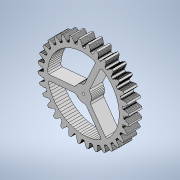
# Autodesk Inventor part: Шестерня 32 зуба
Saved by Autodesk Inventor 2020 (Build 240168000, 168)
## iProperties
Created: 2021-06-13
Part Number: Шестерня 32 зуба
Material: Типовые
Document SubType Name: Modeling
Designer: Антон
Density: 1 g/cm^3
Appearance: По умолчанию
Author: Антон
Autodesk Inventor part; units mm, degrees
(part 1 of 2)
ref_plane "YZ Plane" through (0, 0, 0) normal (1, 0, 0) x (0, 1, 0)
ref_plane "XZ Plane" through (0, 0, 0) normal (0, 1, 0) x (-1, 0, 0)
ref_plane "XY Plane" through (0, 0, 0) normal (0, 0, 1) x (1, 0, 0)
sketch "Эскиз1" plane through (0, 0, 0) normal (0, 0, 1) x (1, 0, 0)
  line L0 (2.3797, 14.7575) -> (2.3075, 14.8611)
  line L1 (2.3075, 14.8611) -> (2.2375, 14.9567)
  line L2 (2.2375, 14.9567) -> (2.1835, 14.9517)
  line L3 (2.1835, 14.9517) -> (2.0746, 14.948)
  line L4 (2.0746, 14.948) -> (1.9648, 14.9497)
  line L5 (1.9648, 14.9497) -> (1.8544, 14.9557)
  line L6 (1.8544, 14.9557) -> (1.6322, 14.9783)
  line L7 (1.6322, 14.9783) -> (1.4083, 15.013)
  line L8 (1.4083, 15.013) -> (1.1833, 15.0583)
  line L9 (1.1833, 15.0583) -> (0.9573, 15.1136)
  line L10 (0.9573, 15.1136) -> (0.7306, 15.178)
  line L11 (0.7306, 15.178) -> (0.5032, 15.2512)
  line L12 (0.5032, 15.2512) -> (0.2756, 15.3329)
  line L13 (0.2756, 15.3329) -> (0.1047, 15.3995)
  line L14 (0.1047, 15.3995) -> (0.0431, 16.0795)
  line L15 (0.0431, 16.0795) -> (0.1992, 16.1757)
  line L16 (0.1992, 16.1757) -> (0.4086, 16.2969)
  line L17 (0.4086, 16.2969) -> (0.619, 16.4098)
  line L18 (0.619, 16.4098) -> (0.8305, 16.5139)
  line L19 (0.8305, 16.5139) -> (1.0429, 16.6088)
  line L20 (1.0429, 16.6088) -> (1.2561, 16.6939)
  line L21 (1.2561, 16.6939) -> (1.4701, 16.7682)
  line L22 (1.4701, 16.7682) -> (1.6846, 16.8303)
  line L23 (1.6846, 16.8303) -> (1.7922, 16.8561)
  line L24 (1.7922, 16.8561) -> (1.8999, 16.8775)
  line L25 (1.8999, 16.8775) -> (2.0077, 16.8934)
  line L26 (2.0077, 16.8934) -> (2.0617, 16.8982)
  line L27 (2.0617, 16.8982) -> (2.1134, 17.0048)
  line L28 (2.1134, 17.0048) -> (2.1657, 17.1197)
  line L29 (2.1657, 17.1197) -> (2.1704, 17.717)
  line L30 (2.1704, 17.717) -> (2.1199, 17.8328)
  line L31 (2.1199, 17.8328) -> (2.0699, 17.9402)
  line L32 (2.0699, 17.9402) -> (2.016, 17.9458)
  line L33 (2.016, 17.9458) -> (1.9084, 17.9634)
  line L34 (1.9084, 17.9634) -> (1.8011, 17.9865)
  line L35 (1.8011, 17.9865) -> (1.694, 18.014)
  line L36 (1.694, 18.014) -> (1.4804, 18.0794)
  line L37 (1.4804, 18.0794) -> (1.2676, 18.1571)
  line L38 (1.2676, 18.1571) -> (1.0557, 18.2455)
  line L39 (1.0557, 18.2455) -> (0.8448, 18.3438)
  line L40 (0.8448, 18.3438) -> (0.635, 18.4512)
  line L41 (0.635, 18.4512) -> (0.4264, 18.5674)
  line L42 (0.4264, 18.5674) -> (0.219, 18.6919)
  line L43 (0.219, 18.6919) -> (0.0644, 18.7905)
  line L44 (0.0644, 18.7905) -> (0.1366, 19.4695)
  line L45 (0.1366, 19.4695) -> (0.3086, 19.5334)
  line L46 (0.3086, 19.5334) -> (0.5375, 19.6114)
  line L47 (0.5375, 19.6114) -> (0.7659, 19.6811)
  line L48 (0.7659, 19.6811) -> (0.9937, 19.7419)
  line L49 (0.9937, 19.7419) -> (1.2205, 19.7936)
  line L50 (1.2205, 19.7936) -> (1.4462, 19.8355)
  line L51 (1.4462, 19.8355) -> (1.6705, 19.8666)
  line L52 (1.6705, 19.8666) -> (1.8932, 19.8857)
  line L53 (1.8932, 19.8857) -> (2.0036, 19.8899)
  line L54 (2.0036, 19.8899) -> (2.1134, 19.8899)
  line L55 (2.1134, 19.8899) -> (2.2223, 19.8845)
  line L56 (2.2223, 19.8845) -> (2.2762, 19.8787)
  line L57 (2.2762, 19.8787) -> (2.3477, 19.9732)
  line L58 (2.3477, 19.9732) -> (2.4214, 20.0756)
  line L59 (2.4214, 20.0756) -> (2.5426, 20.6606)
  line L60 (2.5426, 20.6606) -> (2.5156, 20.7839)
  line L61 (2.5156, 20.7839) -> (2.4875, 20.899)
  line L62 (2.4875, 20.899) -> (2.4357, 20.915)
  line L63 (2.4357, 20.915) -> (2.3336, 20.9533)
  line L64 (2.3336, 20.9533) -> (2.2329, 20.997)
  line L65 (2.2329, 20.997) -> (2.1332, 21.0447)
  line L66 (2.1332, 21.0447) -> (1.9365, 21.1506)
  line L67 (1.9365, 21.1506) -> (1.7429, 21.2683)
  line L68 (1.7429, 21.2683) -> (1.5524, 21.3964)
  line L69 (1.5524, 21.3964) -> (1.3647, 21.5339)
  line L70 (1.3647, 21.5339) -> (1.1799, 21.6802)
  line L71 (1.1799, 21.6802) -> (0.9979, 21.8348)
  line L72 (0.9979, 21.8348) -> (0.8188, 21.9974)
  line L73 (0.8188, 21.9974) -> (0.6864, 22.1243)
  line L74 (0.6864, 22.1243) -> (0.8897, 22.7761)
  line L75 (0.8897, 22.7761) -> (1.0708, 22.8052)
  line L76 (1.0708, 22.8052) -> (1.3106, 22.8371)
  line L77 (1.3106, 22.8371) -> (1.5482, 22.8609)
  line L78 (1.5482, 22.8609) -> (1.7834, 22.8761)
  line L79 (1.7834, 22.8761) -> (2.016, 22.8825)
  line L80 (2.016, 22.8825) -> (2.2456, 22.8795)
  line L81 (2.2456, 22.8795) -> (2.4717, 22.8663)
  line L82 (2.4717, 22.8663) -> (2.6937, 22.8416)
  line L83 (2.6937, 22.8416) -> (2.8029, 22.8242)
  line L84 (2.8029, 22.8242) -> (2.9106, 22.8028)
  line L85 (2.9106, 22.8028) -> (3.0163, 22.7763)
  line L86 (3.0163, 22.7763) -> (3.068, 22.76)
  line L87 (3.068, 22.76) -> (3.1566, 22.8387)
  line L88 (3.1566, 22.8387) -> (3.2489, 22.9249)
  line L89 (3.2489, 22.9249) -> (3.4818, 23.4749)
  line L90 (3.4818, 23.4749) -> (3.4794, 23.6012)
  line L91 (3.4794, 23.6012) -> (3.4743, 23.7196)
  line L92 (3.4743, 23.7196) -> (3.4267, 23.7454)
  line L93 (3.4267, 23.7454) -> (3.334, 23.8028)
  line L94 (3.334, 23.8028) -> (3.2437, 23.8653)
  line L95 (3.2437, 23.8653) -> (3.1553, 23.9316)
  line L96 (3.1553, 23.9316) -> (2.983, 24.0738)
  line L97 (2.983, 24.0738) -> (2.8161, 24.227)
  line L98 (2.8161, 24.227) -> (2.6542, 24.3897)
  line L99 (2.6542, 24.3897) -> (2.497, 24.5612)
  line L100 (2.497, 24.5612) -> (2.3443, 24.7408)
  line L101 (2.3443, 24.7408) -> (2.1959, 24.9279)
  line L102 (2.1959, 24.9279) -> (2.052, 25.1223)
  line L103 (2.052, 25.1223) -> (1.9469, 25.2726)
  line L104 (1.9469, 25.2726) -> (2.2735, 25.8722)
  line L105 (2.2735, 25.8722) -> (2.4568, 25.8655)
  line L106 (2.4568, 25.8655) -> (2.6982, 25.85)
  line L107 (2.6982, 25.85) -> (2.9358, 25.8269)
  line L108 (2.9358, 25.8269) -> (3.1695, 25.796)
  line L109 (3.1695, 25.796) -> (3.3989, 25.7569)
  line L110 (3.3989, 25.7569) -> (3.6234, 25.7092)
  line L111 (3.6234, 25.7092) -> (3.8426, 25.6522)
  line L112 (3.8426, 25.6522) -> (4.0556, 25.5846)
  line L113 (4.0556, 25.5846) -> (4.1593, 25.5462)
  line L114 (4.1593, 25.5462) -> (4.2607, 25.5042)
  line L115 (4.2607, 25.5042) -> (4.3592, 25.4576)
  line L116 (4.3592, 25.4576) -> (4.4068, 25.4315)
  line L117 (4.4068, 25.4315) -> (4.509, 25.4915)
  line L118 (4.509, 25.4915) -> (4.6163, 25.5579)
  line L119 (4.6163, 25.5579) -> (4.9521, 26.052)
  line L120 (4.9521, 26.052) -> (4.9744, 26.1763)
  line L121 (4.9744, 26.1763) -> (4.9925, 26.2934)
  line L122 (4.9925, 26.2934) -> (4.9507, 26.328)
  line L123 (4.9507, 26.328) -> (4.8711, 26.4024)
  line L124 (4.8711, 26.4024) -> (4.7947, 26.4813)
  line L125 (4.7947, 26.4813) -> (4.7209, 26.5636)
  line L126 (4.7209, 26.5636) -> (4.5797, 26.7367)
  line L127 (4.5797, 26.7367) -> (4.4459, 26.9195)
  line L128 (4.4459, 26.9195) -> (4.3189, 27.1107)
  line L129 (4.3189, 27.1107) -> (4.1981, 27.3095)
  line L130 (4.1981, 27.3095) -> (4.0833, 27.5154)
  line L131 (4.0833, 27.5154) -> (3.9744, 27.7279)
  line L132 (3.9744, 27.7279) -> (3.8711, 27.9467)
  line L133 (3.8711, 27.9467) -> (3.7974, 28.1146)
  line L134 (3.7974, 28.1146) -> (4.2346, 28.639)
  line L135 (4.2346, 28.639) -> (4.4131, 28.5966)
  line L136 (4.4131, 28.5966) -> (4.6468, 28.5343)
  line L137 (4.6468, 28.5343) -> (4.8754, 28.4653)
  line L138 (4.8754, 28.4653) -> (5.0986, 28.3894)
  line L139 (5.0986, 28.3894) -> (5.3159, 28.3063)
  line L140 (5.3159, 28.3063) -> (5.5269, 28.2157)
  line L141 (5.5269, 28.2157) -> (5.7307, 28.117)
  line L142 (5.7307, 28.117) -> (5.9264, 28.0092)
  line L143 (5.9264, 28.0092) -> (6.0206, 27.9513)
  line L144 (6.0206, 27.9513) -> (6.1119, 27.8903)
  line L145 (6.1119, 27.8903) -> (6.1994, 27.8254)
  line L146 (6.1994, 27.8254) -> (6.241, 27.7905)
  line L147 (6.241, 27.7905) -> (6.3529, 27.8294)
  line L148 (6.3529, 27.8294) -> (6.4712, 27.8736)
  line L149 (6.4712, 27.8736) -> (6.8968, 28.2927)
  line L150 (6.8968, 28.2927) -> (6.9429, 28.4102)
  line L151 (6.9429, 28.4102) -> (6.9836, 28.5215)
  line L152 (6.9836, 28.5215) -> (6.9494, 28.5636)
  line L153 (6.9494, 28.5636) -> (6.8858, 28.6522)
  line L154 (6.8858, 28.6522) -> (6.8262, 28.7444)
  line L155 (6.8262, 28.7444) -> (6.7699, 28.8395)
  line L156 (6.7699, 28.8395) -> (6.6652, 29.0369)
  line L157 (6.6652, 29.0369) -> (6.5696, 29.2422)
  line L158 (6.5696, 29.2422) -> (6.4824, 29.4546)
  line L159 (6.4824, 29.4546) -> (6.4027, 29.6731)
  line L160 (6.4027, 29.6731) -> (6.3303, 29.8975)
  line L161 (6.3303, 29.8975) -> (6.2649, 30.1272)
  line L162 (6.2649, 30.1272) -> (6.2063, 30.3618)
  line L163 (6.2063, 30.3618) -> (6.1667, 30.5409)
  line L164 (6.1667, 30.5409) -> (6.6979, 30.9699)
  line L165 (6.6979, 30.9699) -> (6.8647, 30.8935)
  line L166 (6.8647, 30.8935) -> (7.0817, 30.7869)
  line L167 (7.0817, 30.7869) -> (7.2925, 30.6746)
  line L168 (7.2925, 30.6746) -> (7.4966, 30.5566)
  line L169 (7.4966, 30.5566) -> (7.6935, 30.4327)
  line L170 (7.6935, 30.4327) -> (7.8827, 30.3027)
  line L171 (7.8827, 30.3027) -> (8.0634, 30.1661)
  line L172 (8.0634, 30.1661) -> (8.2342, 30.0222)
  line L173 (8.2342, 30.0222) -> (8.3154, 29.9471)
  line L174 (8.3154, 29.9471) -> (8.393, 29.8695)
  line L175 (8.393, 29.8695) -> (8.4662, 29.7886)
  line L176 (8.4662, 29.7886) -> (8.5001, 29.7464)
  line L177 (8.5001, 29.7464) -> (8.6175, 29.7626)
  line L178 (8.6175, 29.7626) -> (8.7421, 29.783)
  line L179 (8.7421, 29.783) -> (9.2414, 30.1109)
  line L180 (9.2414, 30.1109) -> (9.3095, 30.2172)
  line L181 (9.3095, 30.2172) -> (9.3711, 30.3185)
  line L182 (9.3711, 30.3185) -> (9.3458, 30.3664)
  line L183 (9.3458, 30.3664) -> (9.3006, 30.4657)
  line L184 (9.3006, 30.4657) -> (9.2603, 30.5677)
  line L185 (9.2603, 30.5677) -> (9.2236, 30.672)
  line L186 (9.2236, 30.672) -> (9.1593, 30.886)
  line L187 (9.1593, 30.886) -> (9.1057, 31.1061)
  line L188 (9.1057, 31.1061) -> (9.0615, 31.3313)
  line L189 (9.0615, 31.3313) -> (9.026, 31.5613)
  line L190 (9.026, 31.5613) -> (8.9988, 31.7954)
  line L191 (8.9988, 31.7954) -> (8.9795, 32.0334)
  line L192 (8.9795, 32.0334) -> (8.9678, 32.275)
  line L193 (8.9678, 32.275) -> (8.9639, 32.4584)
  line L194 (8.9639, 32.4584) -> (9.5686, 32.7755)
  line L195 (9.5686, 32.7755) -> (9.7172, 32.6681)
  line L196 (9.7172, 32.6681) -> (9.9093, 32.5211)
  line L197 (9.9093, 32.5211) -> (10.0941, 32.3698)
  line L198 (10.0941, 32.3698) -> (10.2713, 32.2143)
  line L199 (10.2713, 32.2143) -> (10.4402, 32.0544)
  line L200 (10.4402, 32.0544) -> (10.6004, 31.89)
  line L201 (10.6004, 31.89) -> (10.751, 31.7207)
  line L202 (10.751, 31.7207) -> (10.8905, 31.5463)
  line L203 (10.8905, 31.5463) -> (10.9554, 31.4568)
  line L204 (10.9554, 31.4568) -> (11.0164, 31.3655)
  line L205 (11.0164, 31.3655) -> (11.0724, 31.272)
  line L206 (11.0724, 31.272) -> (11.0975, 31.2239)
  line L207 (11.0975, 31.2239) -> (11.2158, 31.2169)
  line L208 (11.2158, 31.2169) -> (11.342, 31.2126)
  line L209 (11.342, 31.2126) -> (11.8956, 31.4368)
  line L210 (11.8956, 31.4368) -> (11.9832, 31.5278)
  line L211 (11.9832, 31.5278) -> (12.0633, 31.6151)
  line L212 (12.0633, 31.6151) -> (12.0478, 31.667)
  line L213 (12.0478, 31.667) -> (12.0229, 31.7732)
  line L214 (12.0229, 31.7732) -> (12.0032, 31.8812)
  line L215 (12.0032, 31.8812) -> (11.9876, 31.9906)
  line L216 (11.9876, 31.9906) -> (11.9663, 32.213)
  line L217 (11.9663, 32.213) -> (11.9567, 32.4393)
  line L218 (11.9567, 32.4393) -> (11.9573, 32.6689)
  line L219 (11.9573, 32.6689) -> (11.9674, 32.9013)
  line L220 (11.9674, 32.9013) -> (11.9863, 33.1363)
  line L221 (11.9863, 33.1363) -> (12.0138, 33.3735)
  line L222 (12.0138, 33.3735) -> (12.0494, 33.6127)
  line L223 (12.0494, 33.6127) -> (12.0814, 33.7933)
  line L224 (12.0814, 33.7933) -> (12.7363, 33.9864)
  line L225 (12.7363, 33.9864) -> (12.8612, 33.852)
  line L226 (12.8612, 33.852) -> (13.0209, 33.6704)
  line L227 (13.0209, 33.6704) -> (13.1727, 33.486)
  line L228 (13.1727, 33.486) -> (13.316, 33.2989)
  line L229 (13.316, 33.2989) -> (13.4506, 33.1091)
  line L230 (13.4506, 33.1091) -> (13.5756, 32.9166)
  line L231 (13.5756, 32.9166) -> (13.6902, 32.7212)
  line L232 (13.6902, 32.7212) -> (13.793, 32.5228)
  line L233 (13.793, 32.5228) -> (13.8392, 32.4224)
  line L234 (13.8392, 32.4224) -> (13.8813, 32.321)
  line L235 (13.8813, 32.321) -> (13.918, 32.2183)
  line L236 (13.918, 32.2183) -> (13.9332, 32.1663)
  line L237 (13.9332, 32.1663) -> (14.0478, 32.1364)
  line L238 (14.0478, 32.1364) -> (14.1707, 32.1075)
  line L239 (14.1707, 32.1075) -> (14.7575, 32.2194)
  line L240 (14.7575, 32.2194) -> (14.8611, 32.2915)
  line L241 (14.8611, 32.2915) -> (14.9567, 32.3615)
  line L242 (14.9567, 32.3615) -> (14.9517, 32.4155)
  line L243 (14.9517, 32.4155) -> (14.948, 32.5245)
  line L244 (14.948, 32.5245) -> (14.9497, 32.6343)
  line L245 (14.9497, 32.6343) -> (14.9557, 32.7447)
  line L246 (14.9557, 32.7447) -> (14.9783, 32.9669)
  line L247 (14.9783, 32.9669) -> (15.013, 33.1907)
  line L248 (15.013, 33.1907) -> (15.0583, 33.4158)
  line L249 (15.0583, 33.4158) -> (15.1136, 33.6418)
  line L250 (15.1136, 33.6418) -> (15.178, 33.8685)
  line L251 (15.178, 33.8685) -> (15.2512, 34.0958)
  line L252 (15.2512, 34.0958) -> (15.3329, 34.3235)
  line L253 (15.3329, 34.3235) -> (15.3995, 34.4944)
  line L254 (15.3995, 34.4944) -> (16.0795, 34.556)
  line L255 (16.0795, 34.556) -> (16.1757, 34.3998)
  line L256 (16.1757, 34.3998) -> (16.2969, 34.1905)
  line L257 (16.2969, 34.1905) -> (16.4098, 33.9801)
  line L258 (16.4098, 33.9801) -> (16.5139, 33.7686)
  line L259 (16.5139, 33.7686) -> (16.6088, 33.5562)
  line L260 (16.6088, 33.5562) -> (16.6939, 33.343)
  line L261 (16.6939, 33.343) -> (16.7682, 33.129)
  line L262 (16.7682, 33.129) -> (16.8303, 32.9144)
  line L263 (16.8303, 32.9144) -> (16.8561, 32.8069)
  line L264 (16.8561, 32.8069) -> (16.8775, 32.6992)
  line L265 (16.8775, 32.6992) -> (16.8934, 32.5914)
  line L266 (16.8934, 32.5914) -> (16.8982, 32.5374)
  line L267 (16.8982, 32.5374) -> (17.0048, 32.4857)
  line L268 (17.0048, 32.4857) -> (17.1197, 32.4334)
  line L269 (17.1197, 32.4334) -> (17.717, 32.4287)
  line L270 (17.717, 32.4287) -> (17.8328, 32.4792)
  line L271 (17.8328, 32.4792) -> (17.9402, 32.5292)
  line L272 (17.9402, 32.5292) -> (17.9458, 32.5831)
  line L273 (17.9458, 32.5831) -> (17.9634, 32.6907)
  line L274 (17.9634, 32.6907) -> (17.9865, 32.798)
  line L275 (17.9865, 32.798) -> (18.014, 32.9051)
  line L276 (18.014, 32.9051) -> (18.0794, 33.1187)
  line L277 (18.0794, 33.1187) -> (18.1571, 33.3315)
  line L278 (18.1571, 33.3315) -> (18.2455, 33.5433)
  line L279 (18.2455, 33.5433) -> (18.3438, 33.7542)
  line L280 (18.3438, 33.7542) -> (18.4512, 33.9641)
  line L281 (18.4512, 33.9641) -> (18.5674, 34.1727)
  line L282 (18.5674, 34.1727) -> (18.6919, 34.3801)
  line L283 (18.6919, 34.3801) -> (18.7905, 34.5347)
  line L284 (18.7905, 34.5347) -> (19.4695, 34.4624)
  line L285 (19.4695, 34.4624) -> (19.5334, 34.2905)
  line L286 (19.5334, 34.2905) -> (19.6114, 34.0616)
  line L287 (19.6114, 34.0616) -> (19.6811, 33.8332)
  line L288 (19.6811, 33.8332) -> (19.7419, 33.6054)
  line L289 (19.7419, 33.6054) -> (19.7936, 33.3786)
  line L290 (19.7936, 33.3786) -> (19.8355, 33.1529)
  line L291 (19.8355, 33.1529) -> (19.8666, 32.9285)
  line L292 (19.8666, 32.9285) -> (19.8857, 32.7059)
  line L293 (19.8857, 32.7059) -> (19.8899, 32.5954)
  line L294 (19.8899, 32.5954) -> (19.8899, 32.4857)
  line L295 (19.8899, 32.4857) -> (19.8845, 32.3768)
  line L296 (19.8845, 32.3768) -> (19.8787, 32.3229)
  line L297 (19.8787, 32.3229) -> (19.9732, 32.2514)
  line L298 (19.9732, 32.2514) -> (20.0756, 32.1776)
  line L299 (20.0756, 32.1776) -> (20.6606, 32.0565)
  line L300 (20.6606, 32.0565) -> (20.7839, 32.0835)
  line L301 (20.7839, 32.0835) -> (20.899, 32.1116)
  line L302 (20.899, 32.1116) -> (20.915, 32.1634)
  line L303 (20.915, 32.1634) -> (20.9533, 32.2655)
  line L304 (20.9533, 32.2655) -> (20.997, 32.3662)
  line L305 (20.997, 32.3662) -> (21.0447, 32.4659)
  line L306 (21.0447, 32.4659) -> (21.1506, 32.6626)
  line L307 (21.1506, 32.6626) -> (21.2683, 32.8561)
  line L308 (21.2683, 32.8561) -> (21.3964, 33.0467)
  line L309 (21.3964, 33.0467) -> (21.5339, 33.2343)
  line L310 (21.5339, 33.2343) -> (21.6802, 33.4192)
  line L311 (21.6802, 33.4192) -> (21.8348, 33.6011)
  line L312 (21.8348, 33.6011) -> (21.9974, 33.7803)
  line L313 (21.9974, 33.7803) -> (22.1243, 33.9127)
  line L314 (22.1243, 33.9127) -> (22.7761, 33.7093)
  line L315 (22.7761, 33.7093) -> (22.8052, 33.5282)
  line L316 (22.8052, 33.5282) -> (22.8371, 33.2885)
  line L317 (22.8371, 33.2885) -> (22.8609, 33.0509)
  line L318 (22.8609, 33.0509) -> (22.8761, 32.8156)
  line L319 (22.8761, 32.8156) -> (22.8825, 32.5831)
  line L320 (22.8825, 32.5831) -> (22.8795, 32.3535)
  line L321 (22.8795, 32.3535) -> (22.8663, 32.1274)
  line L322 (22.8663, 32.1274) -> (22.8416, 31.9054)
  line L323 (22.8416, 31.9054) -> (22.8242, 31.7962)
  line L324 (22.8242, 31.7962) -> (22.8028, 31.6885)
  line L325 (22.8028, 31.6885) -> (22.7763, 31.5828)
  line L326 (22.7763, 31.5828) -> (22.76, 31.5311)
  line L327 (22.76, 31.5311) -> (22.8387, 31.4425)
  line L328 (22.8387, 31.4425) -> (22.9249, 31.3502)
  line L329 (22.9249, 31.3502) -> (23.4749, 31.1173)
  line L330 (23.4749, 31.1173) -> (23.6012, 31.1197)
  line L331 (23.6012, 31.1197) -> (23.7196, 31.1247)
  line L332 (23.7196, 31.1247) -> (23.7454, 31.1724)
  line L333 (23.7454, 31.1724) -> (23.8028, 31.2651)
  line L334 (23.8028, 31.2651) -> (23.8653, 31.3554)
  line L335 (23.8653, 31.3554) -> (23.9316, 31.4438)
  line L336 (23.9316, 31.4438) -> (24.0738, 31.6161)
  line L337 (24.0738, 31.6161) -> (24.227, 31.783)
  line L338 (24.227, 31.783) -> (24.3897, 31.9449)
  line L339 (24.3897, 31.9449) -> (24.5612, 32.1021)
  line L340 (24.5612, 32.1021) -> (24.7408, 32.2548)
  line L341 (24.7408, 32.2548) -> (24.9279, 32.4031)
  line L342 (24.9279, 32.4031) -> (25.1223, 32.5471)
  line L343 (25.1223, 32.5471) -> (25.2726, 32.6522)
  line L344 (25.2726, 32.6522) -> (25.8722, 32.3256)
  line L345 (25.8722, 32.3256) -> (25.8655, 32.1423)
  line L346 (25.8655, 32.1423) -> (25.85, 31.9009)
  line L347 (25.85, 31.9009) -> (25.8269, 31.6632)
  line L348 (25.8269, 31.6632) -> (25.796, 31.4295)
  line L349 (25.796, 31.4295) -> (25.7569, 31.2002)
  line L350 (25.7569, 31.2002) -> (25.7092, 30.9757)
  line L351 (25.7092, 30.9757) -> (25.6522, 30.7565)
  line L352 (25.6522, 30.7565) -> (25.5846, 30.5435)
  line L353 (25.5846, 30.5435) -> (25.5462, 30.4398)
  line L354 (25.5462, 30.4398) -> (25.5042, 30.3384)
  line L355 (25.5042, 30.3384) -> (25.4576, 30.2399)
  line L356 (25.4576, 30.2399) -> (25.4315, 30.1923)
  line L357 (25.4315, 30.1923) -> (25.4915, 30.0901)
  line L358 (25.4915, 30.0901) -> (25.5579, 29.9827)
  line L359 (25.5579, 29.9827) -> (26.052, 29.647)
  line L360 (26.052, 29.647) -> (26.1763, 29.6247)
  line L361 (26.1763, 29.6247) -> (26.2934, 29.6066)
  line L362 (26.2934, 29.6066) -> (26.328, 29.6483)
  line L363 (26.328, 29.6483) -> (26.4024, 29.728)
  line L364 (26.4024, 29.728) -> (26.4813, 29.8044)
  line L365 (26.4813, 29.8044) -> (26.5636, 29.8782)
  line L366 (26.5636, 29.8782) -> (26.7367, 30.0194)
  line L367 (26.7367, 30.0194) -> (26.9195, 30.1532)
  line L368 (26.9195, 30.1532) -> (27.1107, 30.2802)
  line L369 (27.1107, 30.2802) -> (27.3095, 30.401)
  line L370 (27.3095, 30.401) -> (27.5154, 30.5157)
  line L371 (27.5154, 30.5157) -> (27.7279, 30.6247)
  line L372 (27.7279, 30.6247) -> (27.9467, 30.7279)
  line L373 (27.9467, 30.7279) -> (28.1146, 30.8017)
  line L374 (28.1146, 30.8017) -> (28.639, 30.3644)
  line L375 (28.639, 30.3644) -> (28.5966, 30.186)
  line L376 (28.5966, 30.186) -> (28.5343, 29.9522)
  line L377 (28.5343, 29.9522) -> (28.4653, 29.7236)
  line L378 (28.4653, 29.7236) -> (28.3894, 29.5005)
  line L379 (28.3894, 29.5005) -> (28.3063, 29.2831)
  line L380 (28.3063, 29.2831) -> (28.2157, 29.0722)
  line L381 (28.2157, 29.0722) -> (28.117, 28.8684)
  line L382 (28.117, 28.8684) -> (28.0092, 28.6727)
  line L383 (28.0092, 28.6727) -> (27.9513, 28.5785)
  line L384 (27.9513, 28.5785) -> (27.8903, 28.4872)
  line L385 (27.8903, 28.4872) -> (27.8254, 28.3997)
  line L386 (27.8254, 28.3997) -> (27.7905, 28.3581)
  line L387 (27.7905, 28.3581) -> (27.8294, 28.2462)
  line L388 (27.8294, 28.2462) -> (27.8736, 28.1279)
  line L389 (27.8736, 28.1279) -> (28.2927, 27.7022)
  line L390 (28.2927, 27.7022) -> (28.4102, 27.6561)
  line L391 (28.4102, 27.6561) -> (28.5215, 27.6155)
  line L392 (28.5215, 27.6155) -> (28.5636, 27.6497)
  line L393 (28.5636, 27.6497) -> (28.6522, 27.7133)
  line L394 (28.6522, 27.7133) -> (28.7444, 27.7728)
  line L395 (28.7444, 27.7728) -> (28.8395, 27.8292)
  line L396 (28.8395, 27.8292) -> (29.0369, 27.9339)
  line L397 (29.0369, 27.9339) -> (29.2422, 28.0294)
  line L398 (29.2422, 28.0294) -> (29.4546, 28.1167)
  line L399 (29.4546, 28.1167) -> (29.6731, 28.1964)
  line L400 (29.6731, 28.1964) -> (29.8975, 28.2688)
  line L401 (29.8975, 28.2688) -> (30.1272, 28.3342)
  line L402 (30.1272, 28.3342) -> (30.3618, 28.3928)
  line L403 (30.3618, 28.3928) -> (30.5409, 28.4323)
  line L404 (30.5409, 28.4323) -> (30.9699, 27.9012)
  line L405 (30.9699, 27.9012) -> (30.8935, 27.7344)
  line L406 (30.8935, 27.7344) -> (30.7869, 27.5173)
  line L407 (30.7869, 27.5173) -> (30.6746, 27.3066)
  line L408 (30.6746, 27.3066) -> (30.5566, 27.1025)
  line L409 (30.5566, 27.1025) -> (30.4327, 26.9056)
  line L410 (30.4327, 26.9056) -> (30.3027, 26.7164)
  line L411 (30.3027, 26.7164) -> (30.1661, 26.5357)
  line L412 (30.1661, 26.5357) -> (30.0222, 26.3648)
  line L413 (30.0222, 26.3648) -> (29.9471, 26.2837)
  line L414 (29.9471, 26.2837) -> (29.8695, 26.2061)
  line L415 (29.8695, 26.2061) -> (29.7886, 26.1329)
  line L416 (29.7886, 26.1329) -> (29.7464, 26.0989)
  line L417 (29.7464, 26.0989) -> (29.7626, 25.9816)
  line L418 (29.7626, 25.9816) -> (29.783, 25.857)
  line L419 (29.783, 25.857) -> (30.1109, 25.3577)
  line L420 (30.1109, 25.3577) -> (30.2172, 25.2895)
  line L421 (30.2172, 25.2895) -> (30.3185, 25.228)
  line L422 (30.3185, 25.228) -> (30.3664, 25.2533)
  line L423 (30.3664, 25.2533) -> (30.4657, 25.2984)
  line L424 (30.4657, 25.2984) -> (30.5677, 25.3388)
  line L425 (30.5677, 25.3388) -> (30.672, 25.3755)
  line L426 (30.672, 25.3755) -> (30.886, 25.4397)
  line L427 (30.886, 25.4397) -> (31.1061, 25.4934)
  line L428 (31.1061, 25.4934) -> (31.3313, 25.5376)
  line L429 (31.3313, 25.5376) -> (31.5613, 25.573)
  line L430 (31.5613, 25.573) -> (31.7954, 25.6003)
  line L431 (31.7954, 25.6003) -> (32.0334, 25.6196)
  line L432 (32.0334, 25.6196) -> (32.275, 25.6313)
  line L433 (32.275, 25.6313) -> (32.4584, 25.6352)
  line L434 (32.4584, 25.6352) -> (32.7755, 25.0305)
  line L435 (32.7755, 25.0305) -> (32.6681, 24.8819)
  line L436 (32.6681, 24.8819) -> (32.5211, 24.6898)
  line L437 (32.5211, 24.6898) -> (32.3698, 24.505)
  line L438 (32.3698, 24.505) -> (32.2143, 24.3278)
  line L439 (32.2143, 24.3278) -> (32.0544, 24.1588)
  line L440 (32.0544, 24.1588) -> (31.89, 23.9986)
  line L441 (31.89, 23.9986) -> (31.7207, 23.8481)
  line L442 (31.7207, 23.8481) -> (31.5463, 23.7086)
  line L443 (31.5463, 23.7086) -> (31.4568, 23.6437)
  line L444 (31.4568, 23.6437) -> (31.3655, 23.5827)
  line L445 (31.3655, 23.5827) -> (31.272, 23.5267)
  line L446 (31.272, 23.5267) -> (31.2239, 23.5016)
  line L447 (31.2239, 23.5016) -> (31.2169, 23.3833)
  line L448 (31.2169, 23.3833) -> (31.2126, 23.2571)
  line L449 (31.2126, 23.2571) -> (31.4368, 22.7035)
  line L450 (31.4368, 22.7035) -> (31.5278, 22.6159)
  line L451 (31.5278, 22.6159) -> (31.6151, 22.5358)
  line L452 (31.6151, 22.5358) -> (31.667, 22.5513)
  line L453 (31.667, 22.5513) -> (31.7732, 22.5761)
  line L454 (31.7732, 22.5761) -> (31.8812, 22.5958)
  line L455 (31.8812, 22.5958) -> (31.9906, 22.6115)
  line L456 (31.9906, 22.6115) -> (32.213, 22.6327)
  line L457 (32.213, 22.6327) -> (32.4393, 22.6424)
  line L458 (32.4393, 22.6424) -> (32.6689, 22.6418)
  line L459 (32.6689, 22.6418) -> (32.9013, 22.6317)
  line L460 (32.9013, 22.6317) -> (33.1363, 22.6128)
  line L461 (33.1363, 22.6128) -> (33.3735, 22.5853)
  line L462 (33.3735, 22.5853) -> (33.6127, 22.5496)
  line L463 (33.6127, 22.5496) -> (33.7933, 22.5177)
  line L464 (33.7933, 22.5177) -> (33.9864, 21.8628)
  line L465 (33.9864, 21.8628) -> (33.852, 21.7379)
  line L466 (33.852, 21.7379) -> (33.6704, 21.5782)
  line L467 (33.6704, 21.5782) -> (33.486, 21.4264)
  line L468 (33.486, 21.4264) -> (33.2989, 21.283)
  line L469 (33.2989, 21.283) -> (33.1091, 21.1485)
  line L470 (33.1091, 21.1485) -> (32.9166, 21.0235)
  line L471 (32.9166, 21.0235) -> (32.7212, 20.9088)
  line L472 (32.7212, 20.9088) -> (32.5228, 20.806)
  line L473 (32.5228, 20.806) -> (32.4224, 20.7598)
  line L474 (32.4224, 20.7598) -> (32.321, 20.7178)
  line L475 (32.321, 20.7178) -> (32.2183, 20.6811)
  line L476 (32.2183, 20.6811) -> (32.1663, 20.6659)
  line L477 (32.1663, 20.6659) -> (32.1364, 20.5513)
  line L478 (32.1364, 20.5513) -> (32.1075, 20.4284)
  line L479 (32.1075, 20.4284) -> (32.2194, 19.8416)
  line L480 (32.2194, 19.8416) -> (32.2915, 19.738)
  line L481 (32.2915, 19.738) -> (32.3615, 19.6424)
  line L482 (32.3615, 19.6424) -> (32.4155, 19.6474)
  line L483 (32.4155, 19.6474) -> (32.5245, 19.6511)
  line L484 (32.5245, 19.6511) -> (32.6343, 19.6493)
  line L485 (32.6343, 19.6493) -> (32.7447, 19.6433)
  line L486 (32.7447, 19.6433) -> (32.9669, 19.6208)
  line L487 (32.9669, 19.6208) -> (33.1907, 19.5861)
  line L488 (33.1907, 19.5861) -> (33.4158, 19.5407)
  line L489 (33.4158, 19.5407) -> (33.6418, 19.4855)
  line L490 (33.6418, 19.4855) -> (33.8685, 19.4211)
  line L491 (33.8685, 19.4211) -> (34.0958, 19.3479)
  line L492 (34.0958, 19.3479) -> (34.3235, 19.2662)
  line L493 (34.3235, 19.2662) -> (34.4944, 19.1996)
  line L494 (34.4944, 19.1996) -> (34.556, 18.5196)
  line L495 (34.556, 18.5196) -> (34.3998, 18.4234)
  line L496 (34.3998, 18.4234) -> (34.1905, 18.3022)
  line L497 (34.1905, 18.3022) -> (33.9801, 18.1893)
  line L498 (33.9801, 18.1893) -> (33.7686, 18.0852)
  line L499 (33.7686, 18.0852) -> (33.5562, 17.9903)
  line L500 (33.5562, 17.9903) -> (33.343, 17.9052)
  line L501 (33.343, 17.9052) -> (33.129, 17.8309)
  line L502 (33.129, 17.8309) -> (32.9144, 17.7688)
  line L503 (32.9144, 17.7688) -> (32.8069, 17.743)
  line L504 (32.8069, 17.743) -> (32.6992, 17.7216)
  line L505 (32.6992, 17.7216) -> (32.5914, 17.7056)
  line L506 (32.5914, 17.7056) -> (32.5374, 17.7009)
  line L507 (32.5374, 17.7009) -> (32.4857, 17.5943)
  line L508 (32.4857, 17.5943) -> (32.4334, 17.4794)
  line L509 (32.4334, 17.4794) -> (32.4287, 16.882)
  line L510 (32.4287, 16.882) -> (32.4792, 16.7663)
  line L511 (32.4792, 16.7663) -> (32.5292, 16.6589)
  line L512 (32.5292, 16.6589) -> (32.5831, 16.6533)
  line L513 (32.5831, 16.6533) -> (32.6907, 16.6357)
  line L514 (32.6907, 16.6357) -> (32.798, 16.6125)
  line L515 (32.798, 16.6125) -> (32.9051, 16.5851)
  line L516 (32.9051, 16.5851) -> (33.1187, 16.5196)
  line L517 (33.1187, 16.5196) -> (33.3315, 16.442)
  line L518 (33.3315, 16.442) -> (33.5433, 16.3535)
  line L519 (33.5433, 16.3535) -> (33.7542, 16.2553)
  line L520 (33.7542, 16.2553) -> (33.9641, 16.1479)
  line L521 (33.9641, 16.1479) -> (34.1727, 16.0317)
  line L522 (34.1727, 16.0317) -> (34.3801, 15.9072)
  line L523 (34.3801, 15.9072) -> (34.5347, 15.8085)
  line L524 (34.5347, 15.8085) -> (34.4624, 15.1296)
  line L525 (34.4624, 15.1296) -> (34.2905, 15.0657)
  line L526 (34.2905, 15.0657) -> (34.0616, 14.9876)
  line L527 (34.0616, 14.9876) -> (33.8332, 14.918)
  line L528 (33.8332, 14.918) -> (33.6054, 14.8571)
  line L529 (33.6054, 14.8571) -> (33.3786, 14.8055)
  line L530 (33.3786, 14.8055) -> (33.1529, 14.7636)
  line L531 (33.1529, 14.7636) -> (32.9285, 14.7325)
  line L532 (32.9285, 14.7325) -> (32.7059, 14.7134)
  line L533 (32.7059, 14.7134) -> (32.5954, 14.7092)
  line L534 (32.5954, 14.7092) -> (32.4857, 14.7091)
  line L535 (32.4857, 14.7091) -> (32.3768, 14.7145)
  line L536 (32.3768, 14.7145) -> (32.3229, 14.7204)
  line L537 (32.3229, 14.7204) -> (32.2514, 14.6259)
  line L538 (32.2514, 14.6259) -> (32.1776, 14.5234)
  line L539 (32.1776, 14.5234) -> (32.0565, 13.9385)
  line L540 (32.0565, 13.9385) -> (32.0835, 13.8152)
  line L541 (32.0835, 13.8152) -> (32.1116, 13.7)
  line L542 (32.1116, 13.7) -> (32.1634, 13.684)
  line L543 (32.1634, 13.684) -> (32.2655, 13.6458)
  line L544 (32.2655, 13.6458) -> (32.3662, 13.6021)
  line L545 (32.3662, 13.6021) -> (32.4659, 13.5543)
  line L546 (32.4659, 13.5543) -> (32.6626, 13.4485)
  line L547 (32.6626, 13.4485) -> (32.8561, 13.3308)
  line L548 (32.8561, 13.3308) -> (33.0467, 13.2027)
  line L549 (33.0467, 13.2027) -> (33.2343, 13.0652)
  line L550 (33.2343, 13.0652) -> (33.4192, 12.9189)
  line L551 (33.4192, 12.9189) -> (33.6011, 12.7643)
  line L552 (33.6011, 12.7643) -> (33.7803, 12.6017)
  line L553 (33.7803, 12.6017) -> (33.9127, 12.4748)
  line L554 (33.9127, 12.4748) -> (33.7093, 11.823)
  line L555 (33.7093, 11.823) -> (33.5282, 11.7939)
  line L556 (33.5282, 11.7939) -> (33.2885, 11.762)
  line L557 (33.2885, 11.762) -> (33.0509, 11.7382)
  line L558 (33.0509, 11.7382) -> (32.8156, 11.7229)
  line L559 (32.8156, 11.7229) -> (32.5831, 11.7165)
  line L560 (32.5831, 11.7165) -> (32.3535, 11.7195)
  line L561 (32.3535, 11.7195) -> (32.1274, 11.7327)
  line L562 (32.1274, 11.7327) -> (31.9054, 11.7575)
  line L563 (31.9054, 11.7575) -> (31.7962, 11.7749)
  line L564 (31.7962, 11.7749) -> (31.6885, 11.7962)
  line L565 (31.6885, 11.7962) -> (31.5828, 11.8228)
  line L566 (31.5828, 11.8228) -> (31.5311, 11.8391)
  line L567 (31.5311, 11.8391) -> (31.4425, 11.7603)
  line L568 (31.4425, 11.7603) -> (31.3502, 11.6742)
  line L569 (31.3502, 11.6742) -> (31.1173, 11.1242)
  line L570 (31.1173, 11.1242) -> (31.1197, 10.9979)
  line L571 (31.1197, 10.9979) -> (31.1247, 10.8795)
  line L572 (31.1247, 10.8795) -> (31.1724, 10.8537)
  line L573 (31.1724, 10.8537) -> (31.2651, 10.7963)
  line L574 (31.2651, 10.7963) -> (31.3554, 10.7338)
  line L575 (31.3554, 10.7338) -> (31.4438, 10.6675)
  line L576 (31.4438, 10.6675) -> (31.6161, 10.5253)
  line L577 (31.6161, 10.5253) -> (31.783, 10.3721)
  line L578 (31.783, 10.3721) -> (31.9449, 10.2093)
  line L579 (31.9449, 10.2093) -> (32.1021, 10.0379)
  line L580 (32.1021, 10.0379) -> (32.2548, 9.8583)
  line L581 (32.2548, 9.8583) -> (32.4031, 9.6711)
  line L582 (32.4031, 9.6711) -> (32.5471, 9.4768)
  line L583 (32.5471, 9.4768) -> (32.6522, 9.3264)
  line L584 (32.6522, 9.3264) -> (32.3256, 8.7268)
  line L585 (32.3256, 8.7268) -> (32.1423, 8.7336)
  line L586 (32.1423, 8.7336) -> (31.9009, 8.7491)
  line L587 (31.9009, 8.7491) -> (31.6632, 8.7721)
  line L588 (31.6632, 8.7721) -> (31.4295, 8.8031)
  line L589 (31.4295, 8.8031) -> (31.2002, 8.8421)
  line L590 (31.2002, 8.8421) -> (30.9757, 8.8899)
  line L591 (30.9757, 8.8899) -> (30.7565, 8.9469)
  line L592 (30.7565, 8.9469) -> (30.5435, 9.0145)
  line L593 (30.5435, 9.0145) -> (30.4398, 9.0528)
  line L594 (30.4398, 9.0528) -> (30.3384, 9.0948)
  line L595 (30.3384, 9.0948) -> (30.2399, 9.1415)
  line L596 (30.2399, 9.1415) -> (30.1923, 9.1676)
  line L597 (30.1923, 9.1676) -> (30.0901, 9.1076)
  line L598 (30.0901, 9.1076) -> (29.9827, 9.0411)
  line L599 (29.9827, 9.0411) -> (29.647, 8.5471)
  line L600 (29.647, 8.5471) -> (29.6247, 8.4228)
  line L601 (29.6247, 8.4228) -> (29.6066, 8.3057)
  line L602 (29.6066, 8.3057) -> (29.6483, 8.2711)
  line L603 (29.6483, 8.2711) -> (29.728, 8.1967)
  line L604 (29.728, 8.1967) -> (29.8044, 8.1178)
  line L605 (29.8044, 8.1178) -> (29.8782, 8.0355)
  line L606 (29.8782, 8.0355) -> (30.0194, 7.8624)
  line L607 (30.0194, 7.8624) -> (30.1532, 7.6796)
  line L608 (30.1532, 7.6796) -> (30.2802, 7.4884)
  line L609 (30.2802, 7.4884) -> (30.401, 7.2896)
  line L610 (30.401, 7.2896) -> (30.5157, 7.0837)
  line L611 (30.5157, 7.0837) -> (30.6247, 6.8712)
  line L612 (30.6247, 6.8712) -> (30.7279, 6.6524)
  line L613 (30.7279, 6.6524) -> (30.8017, 6.4845)
  line L614 (30.8017, 6.4845) -> (30.3644, 5.9601)
  line L615 (30.3644, 5.9601) -> (30.186, 6.0025)
  line L616 (30.186, 6.0025) -> (29.9522, 6.0648)
  line L617 (29.9522, 6.0648) -> (29.7236, 6.1338)
  line L618 (29.7236, 6.1338) -> (29.5005, 6.2097)
  line L619 (29.5005, 6.2097) -> (29.2831, 6.2928)
  line L620 (29.2831, 6.2928) -> (29.0722, 6.3834)
  line L621 (29.0722, 6.3834) -> (28.8684, 6.4821)
  line L622 (28.8684, 6.4821) -> (28.6727, 6.5899)
  line L623 (28.6727, 6.5899) -> (28.5785, 6.6478)
  line L624 (28.5785, 6.6478) -> (28.4872, 6.7087)
  line L625 (28.4872, 6.7087) -> (28.3997, 6.7737)
  line L626 (28.3997, 6.7737) -> (28.3581, 6.8086)
  line L627 (28.3581, 6.8086) -> (28.2462, 6.7697)
  line L628 (28.2462, 6.7697) -> (28.1279, 6.7255)
  line L629 (28.1279, 6.7255) -> (27.7022, 6.3064)
  line L630 (27.7022, 6.3064) -> (27.6561, 6.1889)
  line L631 (27.6561, 6.1889) -> (27.6155, 6.0775)
  line L632 (27.6155, 6.0775) -> (27.6497, 6.0354)
  line L633 (27.6497, 6.0354) -> (27.7133, 5.9469)
  line L634 (27.7133, 5.9469) -> (27.7728, 5.8547)
  line L635 (27.7728, 5.8547) -> (27.8292, 5.7595)
  line L636 (27.8292, 5.7595) -> (27.9339, 5.5622)
  line L637 (27.9339, 5.5622) -> (28.0294, 5.3568)
  line L638 (28.0294, 5.3568) -> (28.1167, 5.1445)
  line L639 (28.1167, 5.1445) -> (28.1964, 4.9259)
  line L640 (28.1964, 4.9259) -> (28.2688, 4.7016)
  line L641 (28.2688, 4.7016) -> (28.3342, 4.4719)
  line L642 (28.3342, 4.4719) -> (28.3928, 4.2373)
  line L643 (28.3928, 4.2373) -> (28.4323, 4.0581)
  line L644 (28.4323, 4.0581) -> (27.9012, 3.6292)
  line L645 (27.9012, 3.6292) -> (27.7344, 3.7056)
  line L646 (27.7344, 3.7056) -> (27.5173, 3.8122)
  line L647 (27.5173, 3.8122) -> (27.3066, 3.9245)
  line L648 (27.3066, 3.9245) -> (27.1025, 4.0425)
  line L649 (27.1025, 4.0425) -> (26.9056, 4.1664)
  line L650 (26.9056, 4.1664) -> (26.7164, 4.2964)
  line L651 (26.7164, 4.2964) -> (26.5357, 4.433)
  line L652 (26.5357, 4.433) -> (26.3648, 4.5769)
  line L653 (26.3648, 4.5769) -> (26.2837, 4.652)
  line L654 (26.2837, 4.652) -> (26.2061, 4.7296)
  line L655 (26.2061, 4.7296) -> (26.1329, 4.8105)
  line L656 (26.1329, 4.8105) -> (26.0989, 4.8527)
  line L657 (26.0989, 4.8527) -> (25.9816, 4.8365)
  line L658 (25.9816, 4.8365) -> (25.857, 4.8161)
  line L659 (25.857, 4.8161) -> (25.3577, 4.4882)
  line L660 (25.3577, 4.4882) -> (25.2895, 4.3819)
  line L661 (25.2895, 4.3819) -> (25.228, 4.2806)
  line L662 (25.228, 4.2806) -> (25.2533, 4.2327)
  line L663 (25.2533, 4.2327) -> (25.2984, 4.1334)
  line L664 (25.2984, 4.1334) -> (25.3388, 4.0313)
  line L665 (25.3388, 4.0313) -> (25.3755, 3.9271)
  line L666 (25.3755, 3.9271) -> (25.4397, 3.7131)
  line L667 (25.4397, 3.7131) -> (25.4934, 3.493)
  line L668 (25.4934, 3.493) -> (25.5376, 3.2677)
  line L669 (25.5376, 3.2677) -> (25.573, 3.0378)
  line L670 (25.573, 3.0378) -> (25.6003, 2.8037)
  line L671 (25.6003, 2.8037) -> (25.6196, 2.5657)
  line L672 (25.6196, 2.5657) -> (25.6313, 2.3241)
  line L673 (25.6313, 2.3241) -> (25.6352, 2.1407)
  line L674 (25.6352, 2.1407) -> (25.0305, 1.8236)
  line L675 (25.0305, 1.8236) -> (24.8819, 1.931)
  line L676 (24.8819, 1.931) -> (24.6898, 2.078)
  line L677 (24.6898, 2.078) -> (24.505, 2.2292)
  line L678 (24.505, 2.2292) -> (24.3278, 2.3848)
  line L679 (24.3278, 2.3848) -> (24.1588, 2.5447)
  line L680 (24.1588, 2.5447) -> (23.9986, 2.7091)
  line L681 (23.9986, 2.7091) -> (23.8481, 2.8783)
  line L682 (23.8481, 2.8783) -> (23.7086, 3.0528)
  line L683 (23.7086, 3.0528) -> (23.6437, 3.1423)
  line L684 (23.6437, 3.1423) -> (23.5827, 3.2336)
  line L685 (23.5827, 3.2336) -> (23.5267, 3.3271)
  line L686 (23.5267, 3.3271) -> (23.5016, 3.3752)
  line L687 (23.5016, 3.3752) -> (23.3833, 3.3822)
  line L688 (23.3833, 3.3822) -> (23.2571, 3.3865)
  line L689 (23.2571, 3.3865) -> (22.7035, 3.1623)
  line L690 (22.7035, 3.1623) -> (22.6159, 3.0713)
  line L691 (22.6159, 3.0713) -> (22.5358, 2.984)
  line L692 (22.5358, 2.984) -> (22.5513, 2.932)
  line L693 (22.5513, 2.932) -> (22.5761, 2.8259)
  line L694 (22.5761, 2.8259) -> (22.5958, 2.7179)
  line L695 (22.5958, 2.7179) -> (22.6115, 2.6084)
  line L696 (22.6115, 2.6084) -> (22.6327, 2.3861)
  line L697 (22.6327, 2.3861) -> (22.6424, 2.1598)
  line L698 (22.6424, 2.1598) -> (22.6418, 1.9302)
  line L699 (22.6418, 1.9302) -> (22.6317, 1.6978)
  line L700 (22.6317, 1.6978) -> (22.6128, 1.4628)
  line L701 (22.6128, 1.4628) -> (22.5853, 1.2256)
  line L702 (22.5853, 1.2256) -> (22.5496, 0.9864)
  line L703 (22.5496, 0.9864) -> (22.5177, 0.8057)
  line L704 (22.5177, 0.8057) -> (21.8628, 0.6127)
  line L705 (21.8628, 0.6127) -> (21.7379, 0.7471)
  line L706 (21.7379, 0.7471) -> (21.5782, 0.9287)
  line L707 (21.5782, 0.9287) -> (21.4264, 1.1131)
  line L708 (21.4264, 1.1131) -> (21.283, 1.3002)
  line L709 (21.283, 1.3002) -> (21.1485, 1.49)
  line L710 (21.1485, 1.49) -> (21.0235, 1.6825)
  line L711 (21.0235, 1.6825) -> (20.9088, 1.8779)
  line L712 (20.9088, 1.8779) -> (20.806, 2.0762)
  line L713 (20.806, 2.0762) -> (20.7598, 2.1767)
  line L714 (20.7598, 2.1767) -> (20.7178, 2.2781)
  line L715 (20.7178, 2.2781) -> (20.6811, 2.3807)
  line L716 (20.6811, 2.3807) -> (20.6659, 2.4328)
  line L717 (20.6659, 2.4328) -> (20.5513, 2.4627)
  line L718 (20.5513, 2.4627) -> (20.4284, 2.4916)
  line L719 (20.4284, 2.4916) -> (19.8416, 2.3797)
  line L720 (19.8416, 2.3797) -> (19.738, 2.3075)
  line L721 (19.738, 2.3075) -> (19.6424, 2.2375)
  line L722 (19.6424, 2.2375) -> (19.6474, 2.1835)
  line L723 (19.6474, 2.1835) -> (19.6511, 2.0746)
  line L724 (19.6511, 2.0746) -> (19.6493, 1.9648)
  line L725 (19.6493, 1.9648) -> (19.6433, 1.8544)
  line L726 (19.6433, 1.8544) -> (19.6208, 1.6322)
  line L727 (19.6208, 1.6322) -> (19.5861, 1.4083)
  line L728 (19.5861, 1.4083) -> (19.5407, 1.1833)
  line L729 (19.5407, 1.1833) -> (19.4855, 0.9573)
  line L730 (19.4855, 0.9573) -> (19.4211, 0.7306)
  line L731 (19.4211, 0.7306) -> (19.3479, 0.5032)
  line L732 (19.3479, 0.5032) -> (19.2662, 0.2756)
  line L733 (19.2662, 0.2756) -> (19.1996, 0.1047)
  line L734 (19.1996, 0.1047) -> (18.5196, 0.0431)
  line L735 (18.5196, 0.0431) -> (18.4234, 0.1992)
  line L736 (18.4234, 0.1992) -> (18.3022, 0.4086)
  line L737 (18.3022, 0.4086) -> (18.1893, 0.619)
  line L738 (18.1893, 0.619) -> (18.0852, 0.8305)
  line L739 (18.0852, 0.8305) -> (17.9903, 1.0429)
  line L740 (17.9903, 1.0429) -> (17.9052, 1.2561)
  line L741 (17.9052, 1.2561) -> (17.8309, 1.4701)
  line L742 (17.8309, 1.4701) -> (17.7688, 1.6846)
  line L743 (17.7688, 1.6846) -> (17.743, 1.7922)
  line L744 (17.743, 1.7922) -> (17.7216, 1.8999)
  line L745 (17.7216, 1.8999) -> (17.7056, 2.0077)
  line L746 (17.7056, 2.0077) -> (17.7009, 2.0617)
  line L747 (17.7009, 2.0617) -> (17.5943, 2.1134)
  line L748 (17.5943, 2.1134) -> (17.4794, 2.1657)
  line L749 (17.4794, 2.1657) -> (16.882, 2.1704)
  line L750 (16.882, 2.1704) -> (16.7663, 2.1199)
  line L751 (16.7663, 2.1199) -> (16.6589, 2.0699)
  line L752 (16.6589, 2.0699) -> (16.6533, 2.016)
  line L753 (16.6533, 2.016) -> (16.6357, 1.9084)
  line L754 (16.6357, 1.9084) -> (16.6125, 1.8011)
  line L755 (16.6125, 1.8011) -> (16.5851, 1.694)
  line L756 (16.5851, 1.694) -> (16.5196, 1.4804)
  line L757 (16.5196, 1.4804) -> (16.442, 1.2676)
  line L758 (16.442, 1.2676) -> (16.3535, 1.0557)
  line L759 (16.3535, 1.0557) -> (16.2553, 0.8448)
  line L760 (16.2553, 0.8448) -> (16.1479, 0.635)
  line L761 (16.1479, 0.635) -> (16.0317, 0.4264)
  line L762 (16.0317, 0.4264) -> (15.9072, 0.219)
  line L763 (15.9072, 0.219) -> (15.8085, 0.0644)
  line L764 (15.8085, 0.0644) -> (15.1296, 0.1366)
  line L765 (15.1296, 0.1366) -> (15.0657, 0.3086)
  line L766 (15.0657, 0.3086) -> (14.9876, 0.5375)
  line L767 (14.9876, 0.5375) -> (14.918, 0.7659)
  line L768 (14.918, 0.7659) -> (14.8571, 0.9937)
  line L769 (14.8571, 0.9937) -> (14.8055, 1.2205)
  line L770 (14.8055, 1.2205) -> (14.7636, 1.4462)
  line L771 (14.7636, 1.4462) -> (14.7325, 1.6705)
  line L772 (14.7325, 1.6705) -> (14.7134, 1.8932)
  line L773 (14.7134, 1.8932) -> (14.7092, 2.0036)
  line L774 (14.7092, 2.0036) -> (14.7091, 2.1134)
  line L775 (14.7091, 2.1134) -> (14.7145, 2.2223)
  line L776 (14.7145, 2.2223) -> (14.7204, 2.2762)
  line L777 (14.7204, 2.2762) -> (14.6259, 2.3477)
  line L778 (14.6259, 2.3477) -> (14.5234, 2.4214)
  line L779 (14.5234, 2.4214) -> (13.9385, 2.5426)
  line L780 (13.9385, 2.5426) -> (13.8152, 2.5156)
  line L781 (13.8152, 2.5156) -> (13.7, 2.4875)
  line L782 (13.7, 2.4875) -> (13.684, 2.4357)
  line L783 (13.684, 2.4357) -> (13.6458, 2.3336)
  line L784 (13.6458, 2.3336) -> (13.6021, 2.2329)
  line L785 (13.6021, 2.2329) -> (13.5543, 2.1332)
  line L786 (13.5543, 2.1332) -> (13.4485, 1.9365)
  line L787 (13.4485, 1.9365) -> (13.3308, 1.7429)
  line L788 (13.3308, 1.7429) -> (13.2027, 1.5524)
  line L789 (13.2027, 1.5524) -> (13.0652, 1.3647)
  line L790 (13.0652, 1.3647) -> (12.9189, 1.1799)
  line L791 (12.9189, 1.1799) -> (12.7643, 0.9979)
  line L792 (12.7643, 0.9979) -> (12.6017, 0.8188)
  line L793 (12.6017, 0.8188) -> (12.4748, 0.6864)
  line L794 (12.4748, 0.6864) -> (11.823, 0.8897)
  line L795 (11.823, 0.8897) -> (11.7939, 1.0708)
  line L796 (11.7939, 1.0708) -> (11.762, 1.3106)
  line L797 (11.762, 1.3106) -> (11.7382, 1.5482)
  line L798 (11.7382, 1.5482) -> (11.7229, 1.7834)
  line L799 (11.7229, 1.7834) -> (11.7165, 2.016)
  line L800 (11.7165, 2.016) -> (11.7195, 2.2456)
  line L801 (11.7195, 2.2456) -> (11.7327, 2.4717)
  line L802 (11.7327, 2.4717) -> (11.7575, 2.6937)
  line L803 (11.7575, 2.6937) -> (11.7749, 2.8029)
  line L804 (11.7749, 2.8029) -> (11.7962, 2.9106)
  line L805 (11.7962, 2.9106) -> (11.8228, 3.0163)
  line L806 (11.8228, 3.0163) -> (11.8391, 3.068)
  line L807 (11.8391, 3.068) -> (11.7603, 3.1566)
  line L808 (11.7603, 3.1566) -> (11.6742, 3.2489)
  line L809 (11.6742, 3.2489) -> (11.1242, 3.4818)
  line L810 (11.1242, 3.4818) -> (10.9979, 3.4794)
  line L811 (10.9979, 3.4794) -> (10.8795, 3.4743)
  line L812 (10.8795, 3.4743) -> (10.8537, 3.4267)
  line L813 (10.8537, 3.4267) -> (10.7963, 3.334)
  line L814 (10.7963, 3.334) -> (10.7338, 3.2437)
  line L815 (10.7338, 3.2437) -> (10.6675, 3.1553)
  line L816 (10.6675, 3.1553) -> (10.5253, 2.983)
  line L817 (10.5253, 2.983) -> (10.3721, 2.8161)
  line L818 (10.3721, 2.8161) -> (10.2093, 2.6542)
  line L819 (10.2093, 2.6542) -> (10.0379, 2.497)
  line L820 (10.0379, 2.497) -> (9.8583, 2.3443)
  line L821 (9.8583, 2.3443) -> (9.6711, 2.1959)
  line L822 (9.6711, 2.1959) -> (9.4768, 2.052)
  line L823 (9.4768, 2.052) -> (9.3264, 1.9469)
  line L824 (9.3264, 1.9469) -> (8.7268, 2.2735)
  line L825 (8.7268, 2.2735) -> (8.7336, 2.4568)
  line L826 (8.7336, 2.4568) -> (8.7491, 2.6982)
  line L827 (8.7491, 2.6982) -> (8.7721, 2.9358)
  line L828 (8.7721, 2.9358) -> (8.8031, 3.1695)
  line L829 (8.8031, 3.1695) -> (8.8421, 3.3989)
  line L830 (8.8421, 3.3989) -> (8.8899, 3.6234)
  line L831 (8.8899, 3.6234) -> (8.9469, 3.8426)
  line L832 (8.9469, 3.8426) -> (9.0145, 4.0556)
  line L833 (9.0145, 4.0556) -> (9.0528, 4.1593)
  line L834 (9.0528, 4.1593) -> (9.0948, 4.2607)
  line L835 (9.0948, 4.2607) -> (9.1415, 4.3592)
  line L836 (9.1415, 4.3592) -> (9.1676, 4.4068)
  line L837 (9.1676, 4.4068) -> (9.1076, 4.509)
  line L838 (9.1076, 4.509) -> (9.0411, 4.6163)
  line L839 (9.0411, 4.6163) -> (8.5471, 4.9521)
  line L840 (8.5471, 4.9521) -> (8.4228, 4.9744)
  line L841 (8.4228, 4.9744) -> (8.3057, 4.9925)
  line L842 (8.3057, 4.9925) -> (8.2711, 4.9507)
  line L843 (8.2711, 4.9507) -> (8.1967, 4.8711)
  line L844 (8.1967, 4.8711) -> (8.1178, 4.7947)
  line L845 (8.1178, 4.7947) -> (8.0355, 4.7209)
  line L846 (8.0355, 4.7209) -> (7.8624, 4.5797)
  line L847 (7.8624, 4.5797) -> (7.6796, 4.4459)
  line L848 (7.6796, 4.4459) -> (7.4884, 4.3189)
  line L849 (7.4884, 4.3189) -> (7.2896, 4.1981)
  line L850 (7.2896, 4.1981) -> (7.0837, 4.0833)
  line L851 (7.0837, 4.0833) -> (6.8712, 3.9744)
  line L852 (6.8712, 3.9744) -> (6.6524, 3.8711)
  line L853 (6.6524, 3.8711) -> (6.4845, 3.7974)
  line L854 (6.4845, 3.7974) -> (5.9601, 4.2346)
  line L855 (5.9601, 4.2346) -> (6.0025, 4.4131)
  line L856 (6.0025, 4.4131) -> (6.0648, 4.6468)
  line L857 (6.0648, 4.6468) -> (6.1338, 4.8754)
  line L858 (6.1338, 4.8754) -> (6.2097, 5.0986)
  line L859 (6.2097, 5.0986) -> (6.2928, 5.3159)
  line L860 (6.2928, 5.3159) -> (6.3834, 5.5269)
  line L861 (6.3834, 5.5269) -> (6.4821, 5.7307)
  line L862 (6.4821, 5.7307) -> (6.5899, 5.9264)
  line L863 (6.5899, 5.9264) -> (6.6478, 6.0206)
  line L864 (6.6478, 6.0206) -> (6.7087, 6.1119)
  line L865 (6.7087, 6.1119) -> (6.7737, 6.1994)
  line L866 (6.7737, 6.1994) -> (6.8086, 6.241)
  line L867 (6.8086, 6.241) -> (6.7697, 6.3529)
  line L868 (6.7697, 6.3529) -> (6.7255, 6.4712)
  line L869 (6.7255, 6.4712) -> (6.3064, 6.8968)
  line L870 (6.3064, 6.8968) -> (6.1889, 6.9429)
  line L871 (6.1889, 6.9429) -> (6.0775, 6.9836)
  line L872 (6.0775, 6.9836) -> (6.0354, 6.9494)
  line L873 (6.0354, 6.9494) -> (5.9469, 6.8858)
  line L874 (5.9469, 6.8858) -> (5.8547, 6.8262)
  line L875 (5.8547, 6.8262) -> (5.7595, 6.7699)
  line L876 (5.7595, 6.7699) -> (5.5622, 6.6652)
  line L877 (5.5622, 6.6652) -> (5.3568, 6.5696)
  line L878 (5.3568, 6.5696) -> (5.1445, 6.4824)
  line L879 (5.1445, 6.4824) -> (4.9259, 6.4027)
  line L880 (4.9259, 6.4027) -> (4.7016, 6.3303)
  line L881 (4.7016, 6.3303) -> (4.4719, 6.2649)
  line L882 (4.4719, 6.2649) -> (4.2373, 6.2063)
  line L883 (4.2373, 6.2063) -> (4.0581, 6.1667)
  line L884 (4.0581, 6.1667) -> (3.6292, 6.6979)
  line L885 (3.6292, 6.6979) -> (3.7056, 6.8647)
  line L886 (3.7056, 6.8647) -> (3.8122, 7.0817)
  line L887 (3.8122, 7.0817) -> (3.9245, 7.2925)
  line L888 (3.9245, 7.2925) -> (4.0425, 7.4966)
  line L889 (4.0425, 7.4966) -> (4.1664, 7.6935)
  line L890 (4.1664, 7.6935) -> (4.2964, 7.8827)
  line L891 (4.2964, 7.8827) -> (4.433, 8.0634)
  line L892 (4.433, 8.0634) -> (4.5769, 8.2342)
  line L893 (4.5769, 8.2342) -> (4.652, 8.3154)
  line L894 (4.652, 8.3154) -> (4.7296, 8.393)
  line L895 (4.7296, 8.393) -> (4.8105, 8.4662)
  line L896 (4.8105, 8.4662) -> (4.8527, 8.5001)
  line L897 (4.8527, 8.5001) -> (4.8365, 8.6175)
  line L898 (4.8365, 8.6175) -> (4.8161, 8.7421)
  line L899 (4.8161, 8.7421) -> (4.4882, 9.2414)
  line L900 (4.4882, 9.2414) -> (4.3819, 9.3095)
  line L901 (4.3819, 9.3095) -> (4.2806, 9.3711)
  line L902 (4.2806, 9.3711) -> (4.2327, 9.3458)
  line L903 (4.2327, 9.3458) -> (4.1334, 9.3006)
  line L904 (4.1334, 9.3006) -> (4.0313, 9.2603)
  line L905 (4.0313, 9.2603) -> (3.9271, 9.2236)
  line L906 (3.9271, 9.2236) -> (3.7131, 9.1593)
  line L907 (3.7131, 9.1593) -> (3.493, 9.1057)
  line L908 (3.493, 9.1057) -> (3.2677, 9.0615)
  line L909 (3.2677, 9.0615) -> (3.0378, 9.026)
  line L910 (3.0378, 9.026) -> (2.8037, 8.9988)
  line L911 (2.8037, 8.9988) -> (2.5657, 8.9795)
  line L912 (2.5657, 8.9795) -> (2.3241, 8.9678)
  line L913 (2.3241, 8.9678) -> (2.1407, 8.9639)
  line L914 (2.1407, 8.9639) -> (1.8236, 9.5686)
  line L915 (1.8236, 9.5686) -> (1.931, 9.7172)
  line L916 (1.931, 9.7172) -> (2.078, 9.9093)
  line L917 (2.078, 9.9093) -> (2.2292, 10.0941)
  line L918 (2.2292, 10.0941) -> (2.3848, 10.2713)
  line L919 (2.3848, 10.2713) -> (2.5447, 10.4402)
  line L920 (2.5447, 10.4402) -> (2.7091, 10.6004)
  line L921 (2.7091, 10.6004) -> (2.8783, 10.751)
  line L922 (2.8783, 10.751) -> (3.0528, 10.8905)
  line L923 (3.0528, 10.8905) -> (3.1423, 10.9554)
  line L924 (3.1423, 10.9554) -> (3.2336, 11.0164)
  line L925 (3.2336, 11.0164) -> (3.3271, 11.0724)
  line L926 (3.3271, 11.0724) -> (3.3752, 11.0975)
  line L927 (3.3752, 11.0975) -> (3.3822, 11.2158)
  line L928 (3.3822, 11.2158) -> (3.3865, 11.342)
  line L929 (3.3865, 11.342) -> (3.1623, 11.8956)
  line L930 (3.1623, 11.8956) -> (3.0713, 11.9832)
  line L931 (3.0713, 11.9832) -> (2.984, 12.0633)
  line L932 (2.984, 12.0633) -> (2.932, 12.0478)
  line L933 (2.932, 12.0478) -> (2.8259, 12.0229)
  line L934 (2.8259, 12.0229) -> (2.7179, 12.0032)
  line L935 (2.7179, 12.0032) -> (2.6084, 11.9876)
  line L936 (2.6084, 11.9876) -> (2.3861, 11.9663)
  line L937 (2.3861, 11.9663) -> (2.1598, 11.9567)
  line L938 (2.1598, 11.9567) -> (1.9302, 11.9573)
  line L939 (1.9302, 11.9573) -> (1.6978, 11.9674)
  line L940 (1.6978, 11.9674) -> (1.4628, 11.9863)
  line L941 (1.4628, 11.9863) -> (1.2256, 12.0138)
  line L942 (1.2256, 12.0138) -> (0.9864, 12.0494)
  line L943 (0.9864, 12.0494) -> (0.8057, 12.0814)
  line L944 (0.8057, 12.0814) -> (0.6127, 12.7363)
  line L945 (0.6127, 12.7363) -> (0.7471, 12.8612)
  line L946 (0.7471, 12.8612) -> (0.9287, 13.0209)
  line L947 (0.9287, 13.0209) -> (1.1131, 13.1727)
  line L948 (1.1131, 13.1727) -> (1.3002, 13.316)
  line L949 (1.3002, 13.316) -> (1.49, 13.4506)
  line L950 (1.49, 13.4506) -> (1.6825, 13.5756)
  line L951 (1.6825, 13.5756) -> (1.8779, 13.6902)
  line L952 (1.8779, 13.6902) -> (2.0762, 13.793)
  line L953 (2.0762, 13.793) -> (2.1767, 13.8392)
  line L954 (2.1767, 13.8392) -> (2.2781, 13.8813)
  line L955 (2.2781, 13.8813) -> (2.3807, 13.918)
  line L956 (2.3807, 13.918) -> (2.4328, 13.9332)
  line L957 (2.4328, 13.9332) -> (2.4627, 14.0478)
  line L958 (2.4627, 14.0478) -> (2.4916, 14.1707)
  line L959 (2.4916, 14.1707) -> (2.3797, 14.7575)
  line L960 (14.0444, 15.9625) -> (4.427, 15.0915)
  line L961 (4.427, 15.0915) -> (4.0066, 14.5323)
  line L962 (4.0066, 14.5323) -> (4.2202, 13.6539)
  line L963 (4.2202, 13.6539) -> (4.4918, 12.7917)
  line L964 (4.4918, 12.7917) -> (4.8201, 11.9494)